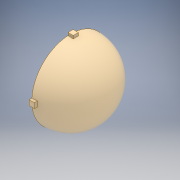
# Autodesk Inventor part: Liner 2
Saved by Autodesk Inventor 2018 (Build 220112000, 112)
## iProperties
Created: 2018-11-29
Part Number: Liner 2
Material: Polyethylene, High Density
Document SubType Name: Modeling
Designer: Ousama
Density: 0.952 g/cm^3
Appearance: Smooth - Off-White
Mass: 4.30046 g
Surface Area: 62.3422 cm^2
Volume: 4.51729 cm^3
Author: Ousama
Autodesk Inventor part; units mm, degrees
sketch "Sketch1" plane through (0, 0, 0) normal (0, 0, 1) x (1, 0, 0)
  line L0 (0, 0) -> (0, 22.5)
  line L1 (0, 22.5) -> (0, 0)
  line L2 (22.5, 0) -> (0, 0)
  arc A0 (22.5, 0) -> (0, 22.5) centre (0, 0) ccw
  dimension "d3" = 22.5
  dimension "d4" = 22.5
  constraints: 6 end point, 2 point on circle, 1 centre point, 1 collinear, 1 perpendicular, 1 vertical
  measures "d3" distance of L0.start L0.end
  measures "d4" radius of A0
revolve "Revolution2" add sketch "Sketch1" angle 360 about axis through (22.5, 0, 0) along (-1, 0, 0)
shell "Shell1" thickness 1.5 removed faces 1 at (0, 7.2821, 1.7949)
ref_plane "Work Plane1" through (0, -24, 0) normal (0, 1, 0) x (-1, 0, 0)
ref_plane "Work Plane2" through (0, 24, 0) normal (0, 1, 0) x (-1, 0, 0)
ref_plane "Work Plane3" through (0, 0, 24) normal (0, 0, 1) x (1, 0, 0)
ref_plane "Work Plane4" through (0, 0, -24) normal (0, 0, 1) x (1, 0, 0)
sketch "Sketch2" plane through (0, 0, 24) normal (0, 0, 1) x (1, 0, 0)
  line L0 (0, -22.5) -> (0, 22.5) projected
  line L1 (0, -1.5) -> (3, -1.5)
  line L2 (3, -1.5) -> (3, 1.5)
  line L3 (3, 1.5) -> (0, 1.5)
  line L4 (0, 1.5) -> (0, -1.5)
  point P0 (0, 0)
  dimension "d24" = 3
  dimension "d25" = 3
  constraints: 8 end point, 2 parallel, 1 horizontal, 1 perpendicular, 1 point on line
  measures "d24" distance of L3.end L2.end
  measures "d25" distance of L2.end L1.end
sketch "Sketch3" plane through (0, -24, 0) normal (0, 1, 0) x (-1, 0, 0)
  line L0 (0, 22.5) -> (0, -22.5) projected
  line L1 (0, -1.5) -> (-3, -1.5)
  line L2 (-3, -1.5) -> (-3, 1.5)
  line L3 (-3, 1.5) -> (0, 1.5)
  line L4 (0, 1.5) -> (0, -1.5)
  point P0 (0, 0)
  dimension "d26" = 3
  dimension "d27" = 3
  constraints: 8 end point, 2 parallel, 1 horizontal, 1 perpendicular, 1 point on line
  measures "d26" distance of L2.end L3.end
  measures "d27" distance of L1.end L2.end
sketch "Sketch4" plane through (0, 0, -24) normal (0, 0, 1) x (1, 0, 0)
  line L0 (0, -22.5) -> (0, 22.5) projected
  line L1 (0, -1.5) -> (3, -1.5)
  line L2 (3, -1.5) -> (3, 1.5)
  line L3 (3, 1.5) -> (0, 1.5)
  line L4 (0, 1.5) -> (0, -1.5)
  point P0 (0, 0)
  dimension "d28" = 3
  dimension "d29" = 3
  constraints: 8 end point, 2 parallel, 1 horizontal, 1 perpendicular, 1 point on line
  measures "d28" distance of L3.end L2.end
  measures "d29" distance of L2.end L1.end
sketch "Sketch5" plane through (0, 24, 0) normal (0, 1, 0) x (-1, 0, 0)
  line L0 (0, -1.4364) -> (-3, -1.4364)
  line L1 (-3, -1.4364) -> (-3, 1.5636)
  line L2 (-3, 1.5636) -> (0, 1.5636)
  line L3 (0, 1.5636) -> (0, -1.4364)
  point P0 (0, 0)
  dimension "d30" = 3
  dimension "d31" = 3
  constraints: 8 end point, 2 parallel, 1 horizontal, 1 perpendicular
  measures "d30" distance of L1.end L2.end
  measures "d31" distance of L0.end L1.end
extrude "Extrusion5" add sketch "Sketch2" against normal up to next
extrude "Extrusion6" add sketch "Sketch3" along normal up to next
extrude "Extrusion7" add sketch "Sketch4" along normal up to next
extrude "Extrusion8" add sketch "Sketch5" against normal up to next
body "Solid2"
